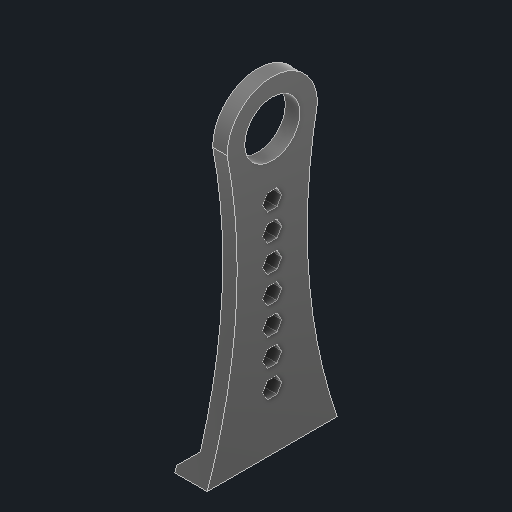
# Autodesk Inventor part: HolderB
Saved by Autodesk Inventor 2023 (Build 270158000, 158)
## iProperties
Created: 2023-11-13
Part Number: HolderB
Material: Acetal Resin, Black
Document SubType Name: Modeling
Designer: danie
Density: 1.425 g/cm^3
Appearance: Smooth - Black
Author: danie
Autodesk Inventor part; units mm, degrees
ref_plane "YZ Plane" through (0, 0, 0) normal (1, 0, 0) x (0, 1, 0)
ref_plane "XZ Plane" through (0, 0, 0) normal (0, 1, 0) x (-1, 0, 0)
ref_plane "XY Plane" through (0, 0, 0) normal (0, 0, 1) x (1, 0, 0)
sketch "Sketch1" plane through (0, 0, 0) normal (1, 0, 0) x (0, 1, 0)
  line L0 (0, 0) -> (155.9349, 0)
  circle A0 centre (155.9349, 0) radius 15.25
  circle A1 centre (155.9349, 0) radius 25
  line L1 (155.6119, 24.9979) -> (0, 35.995)
  line L2 (0, 0) -> (0, 35.995)
  line L3 (155.6119, -24.9979) -> (0, -35.995)
  line L4 (0, 0) -> (0, -35.995)
  arc A2 (0, 35.995) -> (155.6119, 24.9979) centre (98.1634, 318.5597) ccw
  arc A3 (155.6119, -24.9979) -> (0, -35.995) centre (98.1634, -318.5597) ccw
  point P0 (155.6119, -24.9979)
  dimension "d2" = 50
  dimension "d0" = 155.9349
  dimension "d1" = 30.5
  dimension "d3" = 156
  constraints: 10 end point, 4 point on circle, 3 centre point, 3 symmetric about line, 2 coincident, 1 horizontal, 1 vertical, 4 other
  measures "d0" distance of L0.start L0.end
  measures "d1" diameter of A0
  measures "d3" distance of L1.start L1.end
extrude "Extrusion1" add sketch "Sketch1" along normal blind 8 contours L2 A2 A1 L0 | L0 A1 A3 L4 | A1 A2 A3
sketch "Sketch2" plane through (0, 0, 0) normal (-1, 0, 0) x (0, 0, 1)
  arc A0 (24.9979, 155.6119) -> (-24.9979, 155.6119) centre (0, 155.9349) ccw projected
  arc A1 (-35.995, 0) -> (-24.9979, 155.6119) centre (-318.5597, 98.1634) ccw projected
  line L0 (35.995, 0) -> (-35.995, 0) projected
  arc A2 (24.9979, 155.6119) -> (35.995, 0) centre (318.5597, 98.1634) ccw projected
  circle A3 centre (0, 155.9349) radius 15.25 projected
  line L1 (0, 0) -> (0, 13)
  line L2 (0, 13) -> (-31.8089, 13)
  arc A4 (-35.995, 0) -> (-24.9979, 155.6119) centre (-318.5597, 98.1634) ccw projected
  line L3 (0, 13) -> (31.8089, 13)
  arc A5 (24.9979, 155.6119) -> (35.995, 0) centre (318.5597, 98.1634) ccw projected
  point P0 (-31.8089, 13)
  point P1 (31.8089, 13)
  dimension "d6" = 13
  constraints: 6 end point, 2 horizontal, 2 point on circle, 1 vertical
  measures "d6" distance of L1.start L1.end
extrude "Extrusion2" add sketch "Sketch2" along normal blind 10 contours A2 L0 L1 L3 | L2 L1 L0 A1
chamfer "Chamfer1" distance 10 angle 45 1 edges at (-10, 13, 0)
sketch "Sketch3" plane through (0, 0, 0) normal (-1, 0, 0) x (0, 0, 1)
  line L0 (-31.8089, 13) -> (31.8089, 13) projected
  line L1 (0, 13) -> (0, 140.6849)
  circle A0 centre (0, 155.9349) radius 15.25 projected
  line L2 (-5.2273, 76.8425) -> (-2.6137, 81.3695)
  line L3 (-2.6137, 81.3695) -> (2.6137, 81.3695)
  line L4 (2.6137, 81.3695) -> (5.2273, 76.8425)
  line L5 (5.2273, 76.8425) -> (2.6137, 72.3155)
  line L6 (2.6137, 72.3155) -> (-2.6137, 72.3155)
  line L7 (-2.6137, 72.3155) -> (-5.2273, 76.8425)
  line L8 (-5.2273, 91.8425) -> (-2.6137, 96.3695)
  line L9 (-2.6137, 96.3695) -> (2.6137, 96.3695)
  line L10 (2.6137, 96.3695) -> (5.2273, 91.8425)
  line L11 (5.2273, 91.8425) -> (2.6137, 87.3155)
  line L12 (2.6137, 87.3155) -> (-2.6137, 87.3155)
  line L13 (-2.6137, 87.3155) -> (-5.2273, 91.8425)
  line L14 (-5.2273, 106.8425) -> (-2.6137, 111.3695)
  line L15 (-2.6137, 111.3695) -> (2.6137, 111.3695)
  line L16 (2.6137, 111.3695) -> (5.2273, 106.8425)
  line L17 (5.2273, 106.8425) -> (2.6137, 102.3155)
  line L18 (2.6137, 102.3155) -> (-2.6137, 102.3155)
  line L19 (-2.6137, 102.3155) -> (-5.2273, 106.8425)
  line L20 (-5.2273, 121.8425) -> (-2.6137, 126.3695)
  line L21 (-2.6137, 126.3695) -> (2.6137, 126.3695)
  line L22 (2.6137, 126.3695) -> (5.2273, 121.8425)
  line L23 (5.2273, 121.8425) -> (2.6137, 117.3155)
  line L24 (2.6137, 117.3155) -> (-2.6137, 117.3155)
  line L25 (-2.6137, 117.3155) -> (-5.2273, 121.8425)
  line L26 (-2.6137, 66.3695) -> (2.6137, 66.3695)
  line L27 (-5.2273, 61.8425) -> (-2.6137, 66.3695)
  line L28 (2.6137, 66.3695) -> (5.2273, 61.8425)
  line L29 (-2.6137, 57.3155) -> (-5.2273, 61.8425)
  line L30 (5.2273, 61.8425) -> (2.6137, 57.3155)
  line L31 (2.6137, 57.3155) -> (-2.6137, 57.3155)
  line L32 (-2.6137, 51.3695) -> (2.6137, 51.3695)
  line L33 (-5.2273, 46.8425) -> (-2.6137, 51.3695)
  line L34 (2.6137, 51.3695) -> (5.2273, 46.8425)
  line L35 (-2.6137, 42.3155) -> (-5.2273, 46.8425)
  line L36 (5.2273, 46.8425) -> (2.6137, 42.3155)
  line L37 (2.6137, 42.3155) -> (-2.6137, 42.3155)
  line L38 (-2.6137, 36.3695) -> (2.6137, 36.3695)
  line L39 (-5.2273, 31.8425) -> (-2.6137, 36.3695)
  line L40 (2.6137, 36.3695) -> (5.2273, 31.8425)
  line L41 (-2.6137, 27.3155) -> (-5.2273, 31.8425)
  line L42 (5.2273, 31.8425) -> (2.6137, 27.3155)
  line L43 (2.6137, 27.3155) -> (-2.6137, 27.3155)
  line L44 (0, 76.8425) -> (20.7534, 76.8425)
  point P0 (0, 0)
  point P1 (0, 81.3695)
  point P2 (0, 91.8425)
  point P3 (0, 96.3695)
  point P4 (0, 106.8425)
  point P5 (0, 111.3695)
  point P6 (0, 121.8425)
  point P7 (0, 126.3695)
  point P8 (0, 66.3695)
  point P9 (0, 61.8425)
  point P10 (0, 51.3695)
  point P11 (0, 46.8425)
  point P12 (0, 36.3695)
  point P13 (0, 31.8425)
  dimension "d12" = 9.054
  dimension "d15" = 15
  dimension "d22" = 15
  constraints: 88 end point, 3 midpoint, 3 vertical, 1 horizontal, 1 vertical alignment, 98 other
  measures "d12" distance from line of L6 point (0, 81.369)
  measures "d15" distance of L44.start point (0, 91.842)
  measures "d22" distance of L2.end L26.start
extrude "Extrusion3" cut sketch "Sketch3" against normal blind 12 contours L43 L41 L39 L38 L1 | L1 L38 L40 L42 L43 | L24 L25 L20 L21 L1 | L1 L21 L22 L23 L24 | L18 L19 L14 L15 L1 | L1 L15 L16 L17 L18 | L12 L13 L8 L9 L1 | L1 L9 L10 L11 L12 | L6 L7 L2 L3 L1 | L1 L44 L5 L6 | L31 L29 L27 L26 L1 | L1 L26 L28 L30 L31 | L37 L35 L33 L32 L1 | L1 L32 L34 L36 L37 | L1 L3 L4 L44
sketch "Sketch4" plane through (8, 0, -35.995) normal (0, -1, 0) x (1, 0, 0)
  line L0 (-18, 0) -> (0, 0) projected
  line L1 (0, 71.9901) -> (0, 0) projected
  line L2 (-18, 71.9901) -> (0, 71.9901) projected
  line L3 (-18, 0) -> (-18, 71.9901) projected
  line L4 (-18, 71.9901) -> (-9, 71.9901)
  line L5 (-18, 71.9901) -> (-8, 71.9901)
  line L6 (-8, 0) -> (-8, 71.9901)
  line L7 (-8, 67.8039) -> (-8, 55.4246) projected
  line L8 (-13, 71.9901) -> (-13, 0)
  line L9 (-8, 33.3814) -> (0, 33.3814) projected
  line L10 (0, 33.3814) -> (-18, 33.3814)
  line L11 (-13, 71.9901) -> (-13, 33.3814)
  line L12 (-13, 33.3814) -> (-13, 0)
  circle A0 centre (-13, 16.6907) radius 2.5
  circle A1 centre (-13, 52.6857) radius 2.5
  point P0 (-8, 35.995)
  point P1 (-8, 60.9929)
  dimension "d29" = 5
  dimension "d30" = 5
  constraints: 14 end point, 6 point on line, 4 midpoint, 2 centre point, 2 collinear, 2 perpendicular
  measures "d29" diameter of A0
  measures "d30" diameter of A1
extrude "Extrusion4" cut sketch "Sketch4" against normal blind 20 contours A0 L8 | L8 A0 | A1 L8 | L8 A1
chamfer "Chamfer2" distance 2 angle 45 2 edges at (-7.5, 5.5005, -19.3043) (-7.5, 5.5005, 16.6907)
body "Solid1"
